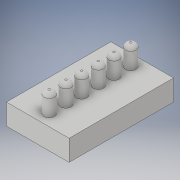
# Autodesk Inventor part: Linien-Sensor
Saved by Autodesk Inventor 2019.5 (Build 235369000, 369)
## iProperties
Created: 2021-09-30
Part Number: Linien-Sensor
Material: Generisch
Document SubType Name: Modeling
Designer: mritt
Density: 1 g/cm^3
Appearance: Vorgabe
Author: mritt
Autodesk Inventor part; units mm, degrees
ref_plane "YZ Plane" through (0, 0, 0) normal (1, 0, 0) x (0, 1, 0)
ref_plane "XZ Plane" through (0, 0, 0) normal (0, 1, 0) x (-1, 0, 0)
ref_plane "XY Plane" through (0, 0, 0) normal (0, 0, 1) x (1, 0, 0)
sketch "Skizze1" plane through (0, 0, 0) normal (0, 1, 0) x (-1, 0, 0)
  line L0 (31.2704, -31.759) -> (1.2704, -31.759)
  line L1 (1.2704, -31.759) -> (1.2704, -81.759)
  line L2 (1.2704, -81.759) -> (31.2704, -81.759)
  line L3 (31.2704, -81.759) -> (31.2704, -31.759)
  point P0 (0, 0)
  dimension "d0" = 50
  dimension "d1" = 30
  constraints: 8 end point, 2 parallel, 1 horizontal, 1 perpendicular
  measures "d0" distance of L2.end L0.start
  measures "d1" distance of L1.end L2.end
extrude "Extrusion1" add sketch "Skizze1" along normal blind 10
sketch "Skizze2" plane through (0, 10, 0) normal (0, 1, 0) x (1, 0, 0)
  circle A0 centre (-16.2704, 37.259) radius 2.5
  circle A1 centre (-16.2704, 60.759) radius 2.5
  circle A2 centre (-16.2704, 76.259) radius 2.5
  circle A3 centre (-16.2704, 45.259) radius 2.5
  circle A4 centre (-16.2704, 52.759) radius 2.5
  circle A5 centre (-16.2704, 68.259) radius 2.5
  line L0 (-31.2704, 81.759) -> (-31.2704, 31.759) projected
  line L1 (-31.2704, 31.759) -> (-1.2704, 31.759) projected
  line L2 (-1.2704, 81.759) -> (-31.2704, 81.759) projected
  point P0 (0, 0)
  dimension "d4" = 5
  dimension "d5" = 5
  dimension "d6" = 5
  dimension "d7" = 5
  dimension "d10" = 5
  dimension "d11" = 5
  dimension "d12" = 15
  dimension "d13" = 15
  dimension "d14" = 15
  dimension "d15" = 15
  dimension "d16" = 15
  dimension "d17" = 15
  dimension "d18" = 8
  dimension "d19" = 8
  dimension "d20" = 8
  dimension "d22" = 5.5
  dimension "d23" = 5.5
  dimension "d24" = 21
  constraints: 6 centre point
  measures "d4" diameter of A0
  measures "d5" diameter of A3
  measures "d6" diameter of A4
  measures "d7" diameter of A1
  measures "d10" diameter of A5
  measures "d11" diameter of A2
  measures "d12" distance from line of A0.centre L0
  measures "d13" distance from line of A3.centre L0
  measures "d14" distance from line of A4.centre L0
  measures "d15" distance from line of A1.centre L0
  measures "d16" distance from line of A5.centre L0
  measures "d17" distance from line of A2.centre L0
  measures "d18" distance of A3.centre A0.centre
  measures "d19" distance of A1.centre A4.centre
  measures "d20" distance of A2.centre A5.centre
  measures "d22" distance from line of A0.centre L1
  measures "d23" distance from line of A2.centre L2
  measures "d24" distance from line of A4.centre L1
extrude "Extrusion2" add sketch "Skizze2" along normal blind 10
fillet "Rundung1" radius 2 6 edges at (-18.7704, 20, -37.259) (-18.7704, 20, -45.259) (-18.7704, 20, -52.759) (-18.7704, 20, -60.759) (-18.7704, 20, -68.259) (-18.7704, 20, -76.259)
